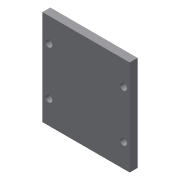
# Autodesk Inventor part: top
Saved by Autodesk Inventor 2015 (Build 190159000, 159)
## iProperties
Created: 2016-11-07
Part Number: top
Material: Generic
Document SubType Name: Modeling
Designer: HAL9000
Density: 1 g/cm^3
Appearance: Default
Author: HAL9000
Autodesk Inventor part; units mm, degrees
ref_plane "YZ Plane" through (0, 0, 0) normal (1, 0, 0) x (0, 1, 0)
ref_plane "XZ Plane" through (0, 0, 0) normal (0, 1, 0) x (-1, 0, 0)
ref_plane "XY Plane" through (0, 0, 0) normal (0, 0, 1) x (1, 0, 0)
sketch "Sketch1" plane through (0, 0, 0) normal (0, 0, 1) x (1, 0, 0)
  line L0 (0, 0) -> (69.85, 0)
  line L1 (69.85, 0) -> (69.85, 76.2)
  line L2 (69.85, 76.2) -> (0, 76.2)
  line L3 (0, 76.2) -> (0, 0)
  line L4 (0, 0) -> (5.08, 0)
  line L5 (5.08, 0) -> (5.08, 19.05)
  line L6 (5.08, 19.05) -> (5.08, 38.1)
  line L7 (5.08, 38.1) -> (5.08, 57.15)
  line L8 (69.85, 0) -> (64.77, 0)
  line L9 (64.77, 0) -> (64.77, 19.05)
  line L10 (64.77, 19.05) -> (64.77, 38.1)
  line L11 (64.77, 38.1) -> (64.77, 57.15)
  dimension "d0" = 69.85
  dimension "d1" = 76.2
  dimension "d2" = 5.08
  dimension "d3" = 19.05
  dimension "d4" = 19.05
  dimension "d5" = 19.05
  dimension "d6" = 5.08
  dimension "d7" = 19.05
  dimension "d8" = 19.05
  dimension "d9" = 19.05
  constraints: 24 end point, 6 point on line, 5 perpendicular, 1 horizontal
  measures "d0" distance of L0.start L0.end
  measures "d1" distance of L0.end L1.end
  measures "d2" distance of L0.start L4.end
  measures "d3" distance of L4.end L5.end
  measures "d4" distance of L5.end L6.end
  measures "d5" distance of L6.end L7.end
  measures "d6" distance of L0.end L8.end
  measures "d7" distance of L8.end L9.end
  measures "d8" distance of L9.end L10.end
  measures "d9" distance of L10.end L11.end
extrude "Extrusion1" add sketch "Sketch1" along normal blind 6.35
sketch "Sketch2" plane through (0, 0, 6.35) normal (0, 0, 1) x (1, 0, 0)
  line L0 (0, 0) -> (5.08, 0)
  line L1 (0, 0) -> (69.85, 0) projected
  line L2 (69.85, 0) -> (64.77, 0)
  line L3 (5.08, 0) -> (5.08, 19.05)
  line L4 (64.77, 0) -> (64.77, 19.05)
  point P0 (5.08, 57.15)
  point P1 (64.77, 57.15)
  dimension "d12" = 5.08
  dimension "d13" = 5.08
  dimension "d14" = 19.05
  dimension "d17" = 19.05
  constraints: 8 end point, 4 coincident, 2 point on line
  measures "d12" distance of L0.start L0.end
  measures "d13" distance of L1.end L2.end
  measures "d14" distance of L0.end L3.end
  measures "d17" distance of L2.end L4.end
hole "Hole1" at (5.08, 57.15, 6.35) at (5.08, 19.05, 6.35) at (64.77, 19.05, 6.35) at (64.77, 57.15, 6.35) direction (0, 0, -1) diameter 4.3656 depth 25.4 tip angle 118
sketch "Sketch3" plane through (0, 0, 6.35) normal (0, 0, 1) x (1, 0, 0)
  circle A0 centre (64.77, 19.05) radius 2.1828 projected
  circle A1 centre (5.08, 57.15) radius 2.1828 projected
  circle A2 centre (5.08, 19.05) radius 2.1828 projected
  circle A3 centre (64.77, 57.15) radius 2.1828 projected
  line L0 (0, 0) -> (69.85, 0) projected
  line L1 (69.85, 0) -> (69.85, 76.2) projected
  line L2 (69.85, 76.2) -> (0, 76.2) projected
  line L3 (0, 76.2) -> (0, 0) projected
  constraints: 4 coincident
hole "Hole2" at (5.08, 57.15, 6.35) at (5.08, 19.05, 6.35) at (64.77, 19.05, 6.35) at (64.77, 57.15, 6.35) direction (0, 0, -1) diameter 5.7404 depth 3.556 tip angle 118
body "Solid1"
